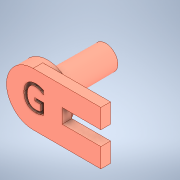
# Autodesk Inventor part: innerGear_1
Saved by Autodesk Inventor 2020.1 (Build 241239000, 239)
## iProperties
Created: 2020-01-18
Part Number: innerGear_1
Material: Generic
Document SubType Name: Modeling
Designer: Ali
Density: 1 g/cm^3
Appearance: Default
Author: Ali
Autodesk Inventor part; units mm, degrees
ref_plane "YZ Plane" through (0, 0, 0) normal (1, 0, 0) x (0, 1, 0)
ref_plane "XZ Plane" through (0, 0, 0) normal (0, 1, 0) x (-1, 0, 0)
ref_plane "XY Plane" through (0, 0, 0) normal (0, 0, 1) x (1, 0, 0)
sketch "Sketch1" plane through (0, 0, 0) normal (0, 0, 1) x (1, 0, 0)
  circle A0 centre (0, 0) radius 5
  dimension "d0" = 10
  constraints: 1 centre point, 1 coincident
  measures "d0" diameter of A0
extrude "Extrusion1" add sketch "Sketch1" along normal blind 1
sketch "Sketch2" plane through (0, 0, 1) normal (0, 0, 1) x (1, 0, 0)
  circle A0 centre (0, 0) radius 1.25
  dimension "d3" = 2.5
  constraints: 1 centre point, 1 coincident
  measures "d3" diameter of A0
extrude "Extrusion2" add sketch "Sketch2" along normal blind 10
ref_plane "Work Plane1" through (0, 0, 5) normal (0, 0, 1) x (1, 0, 0)
sketch "Sketch4" plane through (0, 0, 5) normal (0, 0, 1) x (1, 0, 0)
  circle A0 centre (0, 0) radius 1.25 projected
  circle A1 centre (0, 0) radius 2.75
  dimension "d14" = 1.5
  constraints: 1 centre point
  measures "d14" radial gap between concentric circles of A0 A1
extrude "Extrusion4" add sketch "Sketch4" against normal blind 0.5
sketch "Sketch5" plane through (0, 0, 4.5) normal (0, 0, -1) x (-1, 0, 0)
  circle A0 centre (0, 0) radius 2.75 projected
  line L0 (0, 2.75) -> (0, -2.75) construction
  line L1 (0, -2.75) -> (7, -2.75)
  line L2 (7, -2.75) -> (7, 2.75)
  line L3 (7, 2.75) -> (0, 2.75)
  line L4 (0, 2.75) -> (0, -2.75)
  dimension "d18" = 7
  constraints: 10 end point, 2 parallel, 2 point on circle, 1 horizontal, 1 perpendicular, 1 vertical
  measures "d18" distance of L0.end L1.end
extrude "Extrusion5" add sketch "Sketch5" along normal blind 1
sketch "Sketch6" plane through (0, 0, 3.5) normal (0, 0, -1) x (-1, 0, 0)
  line L0 (7, -2.75) -> (7, 2.75) projected
  line L1 (7, 2.75) -> (0, 2.75) projected
  arc A0 (0, 2.75) -> (0, -2.75) centre (0, 0) ccw projected
  line L2 (0, -2.75) -> (7, -2.75) projected
  circle A1 centre (0, 0) radius 1.25 projected
  line L3 (7, 0) -> (5.7457, 0) construction
  line L4 (7, -2.75) -> (7, 2.75) projected
  line L5 (7, -0.75) -> (3, -0.75)
  line L6 (3, -0.75) -> (3, 0.75)
  line L7 (3, 0.75) -> (7, 0.75)
  line L8 (7, 0.75) -> (7, -0.75)
  point P0 (7, 0.75)
  dimension "d21" = 1.5
  dimension "d22" = 0.75
  dimension "d23" = 4
  constraints: 10 end point, 2 horizontal, 2 parallel, 1 midpoint, 1 perpendicular, 1 point on line
  measures "d21" distance of L5.end L6.end
  measures "d22" distance between parallel lines of L3 L7
  measures "d23" distance of L6.end L7.end
extrude "Extrusion6" cut sketch "Sketch6" against normal up to surface (1 mm away) contours L5 L6 L7 L0
draft "FaceDraft2" angle 0.5 pull direction (0, 0, 1) faces at (1.2459, -0.1006, 9) fixed edges at (-1.25, 0, 11)
sketch "Sketch8" plane through (0, 0, 3.5) normal (0, 0, -1) x (-1, 0, 0)
  line L0 (3, 0.75) -> (7, 0.75) projected
  line L1 (7, 0.75) -> (7, 2.75) projected
  line L2 (7, 2.75) -> (0, 2.75) projected
  arc A0 (0, 2.75) -> (0, -2.75) centre (0, 0) ccw projected
  line L3 (0, -2.75) -> (7, -2.75) projected
  line L4 (7, -2.75) -> (7, -0.75) projected
  line L5 (7, -0.75) -> (3, -0.75) projected
  line L6 (3, -0.75) -> (3, 0.75) projected
  circle A1 centre (0, 0) radius 1.25 projected
extrude "Extrusion8" cut sketch "Sketch8" along normal blind 25.4 contours L6 L5 L4 L3 A0 L2 L1 L0 | A1
sketch "Sketch9" plane through (0, 0, 0) normal (0, 0, -1) x (-1, 0, 0)
  line L0 (4.1758, -2.75) -> (0, -2.75) projected
  arc A0 (0, 2.75) -> (0, -2.75) centre (0, 0) ccw projected
  line L1 (0, 2.75) -> (4.1758, 2.75) projected
  arc A1 (4.1758, 2.75) -> (4.1758, -2.75) centre (0, 0) ccw projected
  line L2 (3, -0.75) -> (4.9434, -0.75) projected
  arc A2 (4.9434, -0.75) -> (4.9434, 0.75) centre (0, 0) ccw projected
  line L3 (4.9434, 0.75) -> (3, 0.75) projected
  line L4 (3, 0.75) -> (3, -0.75) projected
extrude "Extrusion9" cut sketch "Sketch9" against normal up to surface (1 mm away)
sketch "Sketch10" plane through (0, 0, 3.5) normal (0, 0, -1) x (-1, 0, 0)
  line L0 (-1.0676, 1.5273) -> (1.7309, 1.5273) construction
  line L1 (1.7309, 1.5273) -> (1.7309, -1.6344) construction
  line L2 (1.7309, -1.6344) -> (-1.0676, -1.6344) construction
  line L3 (-1.0676, -1.6344) -> (-1.0676, 1.5273) construction
  spline S0 degree 2 poles (0.2539, -1.1074) (-0.0158, -1.1074) (-0.4624, -0.9428) (-0.623, -0.776) knots 0 0 0 1 2 2 2
  spline S1 degree 2 poles (-0.623, -0.776) (-0.7835, -0.6073) (-0.9544, -0.1091) (-0.9544, 0.214) knots 0 0 0 1 2 2 2
  spline S2 degree 2 poles (-0.9544, 0.214) (-0.9544, 0.5207) (-0.7815, 1.0065) (-0.6209, 1.1794) knots 0 0 0 1 2 2 2
  spline S3 degree 2 poles (-0.6209, 1.1794) (-0.4666, 1.3461) (-0.0137, 1.5273) (0.2559, 1.5273) knots 0 0 0 1 2 2 2
  spline S4 degree 2 poles (0.2559, 1.5273) (0.3856, 1.5273) (0.6202, 1.4902) (0.7273, 1.4573) knots 0 0 0 1 2 2 2
  spline S5 degree 2 poles (0.7273, 1.4573) (0.8137, 1.4326) (1.0237, 1.342) (1.0875, 1.3091) knots 0 0 0 1 2 2 2
  line L4 (1.0875, 1.3091) -> (1.0875, 0.9015)
  line L5 (1.0875, 0.9015) -> (1.0587, 0.9015)
  spline S6 degree 2 poles (1.0587, 0.9015) (0.9949, 0.9571) (0.8611, 1.058) (0.7376, 1.1156) knots 0 0 0 1 2 2 2
  spline S7 degree 2 poles (0.7376, 1.1156) (0.6347, 1.167) (0.3691, 1.235) (0.2168, 1.235) knots 0 0 0 1 2 2 2
  spline S8 degree 2 poles (0.2168, 1.235) (-0.1496, 1.235) (-0.6024, 0.6833) (-0.6024, 0.2243) knots 0 0 0 1 2 2 2
  spline S9 degree 2 poles (-0.6024, 0.2243) (-0.6024, -0.0309) (-0.483, -0.4138) (-0.3698, -0.5455) knots 0 0 0 1 2 2 2
  spline S10 degree 2 poles (-0.3698, -0.5455) (-0.2607, -0.6772) (0.048, -0.8151) (0.2415, -0.8151) knots 0 0 0 1 2 2 2
  spline S11 degree 2 poles (0.2415, -0.8151) (0.3835, -0.8151) (0.6676, -0.774) (0.7643, -0.7328) knots 0 0 0 1 2 2 2
  line L6 (0.7643, -0.7328) -> (0.7643, -0.0762)
  line L7 (0.7643, -0.0762) -> (0.1756, -0.0762)
  line L8 (0.1756, -0.0762) -> (0.1756, 0.2202)
  line L9 (0.1756, 0.2202) -> (1.0978, 0.2202)
  line L10 (1.0978, 0.2202) -> (1.0978, -0.8892)
  spline S12 degree 2 poles (1.0978, -0.8892) (1.034, -0.9181) (0.8158, -1.0066) (0.7232, -1.0333) knots 0 0 0 1 2 2 2
  spline S13 degree 2 poles (0.7232, -1.0333) (0.5976, -1.0704) (0.3959, -1.1074) (0.2539, -1.1074) knots 0 0 0 1 2 2 2
  point P0 (0, 0)
  constraints: 2 other
emboss "Emboss1" sketch "Sketch10" operation cut depth 1.27 direction (0, 0, 1)
equation "\"d1\" = IG_gearThickness"
equation "\"d3\" = IG_shaftDiameter"
equation "\"d4\" = IG_shaftLength"
equation "\"d14\" = IG_skirtOffset"
equation "\"d15\" = IG_skirtThickness"
equation "\"d18\" = IG_extentionLength"
equation "\"d19\" = IG_extentionThickness"
equation "\"d21\" = IG_slitWidth"
equation "\"d22\" = 0.5 * d21"
equation "\"d23\" = IG_slitlength"
equation "\"LE_thickness\" = 2"
equation "\"TempSpotReserved19\" = 0"
equation "\"Wheel_Related_W_\" = 0"
equation "\"W_innerDiameter\" = 35"
equation "\"W_innerDepth\" = 4.5"
equation "\"W_wallThickness\" = 1"
equation "\"W_holesClearance\" = 0.3"
equation "\"W_outerGearHoleDiameter\" = 2.1"
equation "\"W_innerGearHoleDiameter\" = 5.1"
equation "\"TempSpotReserved7\" = 0"
equation "\"TempSpotReserved8\" = 0"
equation "\"TempSpotReserved9\" = 0"
equation "\"TempSpotReserved10\" = 0"
equation "\"TempSpotReserved11\" = 0"
equation "\"TempSpotReserved12\" = 0"
equation "\"TempSpotReserved13\" = 0"
equation "\"TempSpotReserved14\" = 0"
equation "\"TempSpotReserved15\" = 0"
equation "\"TempSpotReserved16\" = 0"
equation "\"TempSpotReserved17\" = 0"
equation "\"TempSpotReserved18\" = 0"
equation "\"TempSpotReserved20\" = 0"
equation "\"Inner_Gear_Related_IG_\" = 0"
equation "\"IG_shaftDiameter\" = 2.5"
equation "\"IG_shaftLength\" = 10"
equation "\"IG_gearThickness\" = 1"
equation "\"TempSpotReserved25\" = 0"
equation "\"TempSpotReserved26\" = 0"
equation "\"TempSpotReserved27\" = 0"
equation "\"TempSpotReserved28\" = 0"
equation "\"TempSpotReserved29\" = 0"
equation "\"TempSpotReserved30\" = 0"
equation "\"TempSpotReserved31\" = 0"
equation "\"TempSpotReserved32\" = 0"
equation "\"TempSpotReserved33\" = 0"
equation "\"TempSpotReserved34\" = 0"
equation "\"TempSpotReserved35\" = 0"
equation "\"TempSpotReserved36\" = 0"
equation "\"TempSpotReserved37\" = 0"
equation "\"TempSpotReserved38\" = 0"
equation "\"TempSpotReserved39\" = 0"
equation "\"TempSpotReserved40\" = 0"
equation "\"Outer_Gear_Related_OG_\" = 0"
equation "\"OG_shaftDiameter\" = 1.5"
equation "\"OG_shaftLength\" = 5"
equation "\"OG_gearThickness\" = 1"
equation "\"TempSpotReserved47\" = 0"
equation "\"TempSpotReserved48\" = 0"
equation "\"TempSpotReserved49\" = 0"
equation "\"TempSpotReserved50\" = 0"
equation "\"TempSpotReserved51\" = 0"
equation "\"TempSpotReserved52\" = 0"
equation "\"TempSpotReserved53\" = 0"
equation "\"TempSpotReserved54\" = 0"
equation "\"TempSpotReserved55\" = 0"
equation "\"TempSpotReserved56\" = 0"
equation "\"TempSpotReserved57\" = 0"
equation "\"TempSpotReserved58\" = 0"
equation "\"TempSpotReserved59\" = 0"
equation "\"TempSpotReserved60\" = 0"
equation "\"Leg_Extensions_Related_LE_\" = 0"
equation "\"LE_baseDiameter\" = 2"
equation "\"LE_maxLength\" = 10.64459"
equation "\"B_bearingThickness\" = 1"
equation "\"TempSpotReserved43\" = 0"
equation "\"TempSpotReserved45\" = 0"
equation "\"Thisisatest\" = 25.4"
equation "\"TempSpotReserved46\" = 0"
equation "\"TempSpotReserved44\" = 0"
equation "\"LE_offsetAboveOuterGear\" = 0"
equation "\"Bearing_Related_B_\" = 0"
equation "\"TempSpotReserved42\" = 0"
equation "\"OG_skirtOffset\" = 1"
equation "\"OG_skirtThickness\" = 1"
equation "\"IG_skirtThickness\" = 0.5"
equation "\"IG_skirtOffset\" = 1.5"
equation "\"d13\" = OG_shaftLength - W_wallThickness"
equation "\"IG_extentionLength\" = 7"
equation "\"IG_extentionThickness\" = 1"
equation "\"IG_slitWidth\" = 1.5"
equation "\"IG_slitlength\" = 4"
equation "\"IG_slitClearance\" = 0.3"
body "Solid1"
